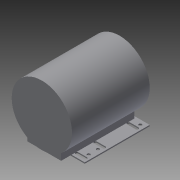
# Autodesk Inventor part: Motor4
Saved by Autodesk Inventor 2016 (Build 200138000, 138)
## iProperties
Created: 2016-02-24
Part Number: Motor4
Material: Generic
Document SubType Name: Modeling
Designer: jonesdm
Density: 1 g/cm^3
Appearance: Default
Author: jonesdm
Autodesk Inventor part; units mm, degrees
ref_plane "YZ Plane" through (0, 0, 0) normal (1, 0, 0) x (0, 1, 0)
ref_plane "XZ Plane" through (0, 0, 0) normal (0, 1, 0) x (-1, 0, 0)
ref_plane "XY Plane" through (0, 0, 0) normal (0, 0, 1) x (1, 0, 0)
sketch "Sketch1" plane through (0, 0, 0) normal (0, 0, 1) x (1, 0, 0)
  circle A0 centre (0, 0) radius 7.9375
  line L0 (-2.4257, 7.5578) -> (-2.4257, 10.0978)
  line L1 (-2.4257, 10.0978) -> (2.4257, 10.0978)
  line L2 (2.4257, 10.0978) -> (2.4257, 7.5578)
  point P0 (0, 10.0978)
  dimension "d0" = 15.875
  dimension "d1" = 2.54
  dimension "d2" = 4.8514
  constraints: 6 end point, 2 point on circle, 1 centre point, 1 coincident, 1 horizontal, 1 midpoint, 1 perpendicular, 1 vertical, 1 vertical alignment
  measures "d0" diameter of A0
  measures "d1" distance of L1.end L2.end
  measures "d2" distance of L0.end L1.end
extrude "Extrusion1" add sketch "Sketch1" along normal blind 50.8
sketch "Sketch2" plane through (0, 0, 50.8) normal (0, 0, 1) x (1, 0, 0)
  circle A0 centre (0, 0) radius 82.55
  dimension "d5" = 165.1
  constraints: 1 centre point, 1 coincident
  measures "d5" diameter of A0
extrude "Extrusion2" add sketch "Sketch2" along normal blind 212.7758
sketch "Sketch3" plane through (0, 0, 50.8) normal (0, 0, -1) x (-1, 0, 0)
  circle A0 centre (0, 0) radius 73.025
  arc A1 (-2.4257, 7.5578) -> (2.4257, 7.5578) centre (0, 0) ccw projected
  line L0 (0, 0) -> (51.6365, 51.6365)
  line L1 (0, 0) -> (73.025, 0) construction
  line L2 (0, 0) -> (51.6365, -51.6365)
  line L3 (0, 0) -> (73.025, 0) construction
  line L4 (0, 0) -> (-51.6365, 51.6365)
  line L5 (0, 0) -> (73.025, 0) construction
  line L6 (0, 0) -> (-51.6365, -51.6365)
  line L7 (0, 0) -> (73.025, 0) construction
  dimension "d8" = 146.05
  dimension "d9" = 45
  dimension "d10" = 45
  dimension "d11" = 135
  dimension "d12" = 135
  constraints: 16 end point, 5 coincident, 4 equal length, 4 horizontal, 4 point on circle, 1 centre point
  measures "d8" diameter of A0
  measures "d9" angle of L1 L0
  measures "d10" angle of L2 L3
  measures "d11" angle of L5 L4
  measures "d12" angle of L6 L7
hole "Hole1" at (51.6365, 51.6365, 50.8) at (-51.6365, 51.6365, 50.8) at (-51.6365, -51.6365, 50.8) at (51.6365, -51.6365, 50.8) direction (0, 0, 1) diameter 4.9784 depth 19.05 tip angle 118 thread size "1/4-20 UNC" class "2B" standard "ANSI Unified Screw Threads"
ref_plane "Work Plane2" through (0, -82.55, 50.8) normal (0, 1, 0) x (-1, 0, 0)
sketch "Sketch4" plane through (0, -82.55, 50.8) normal (0, 1, 0) x (-1, 0, 0)
  line L0 (82.55, 212.7758) -> (-82.55, 212.7758) projected
  line L1 (-82.55, 0) -> (82.55, 0) projected
  line L2 (82.55, 0) -> (82.55, 177.8) projected
  line L3 (-82.55, 0) -> (-82.55, 177.8) projected
  line L4 (-46.355, 6.35) -> (46.355, 6.35)
  line L5 (46.355, 6.35) -> (46.355, 206.4258)
  line L6 (46.355, 206.4258) -> (-46.355, 206.4258)
  line L7 (-46.355, 206.4258) -> (-46.355, 6.35)
  point P0 (0, -50.8)
  point P1 (0, 6.35)
  dimension "d20" = 200.0758
  dimension "d21" = 6.35
  dimension "d22" = 92.71
  constraints: 8 end point, 2 parallel, 1 horizontal, 1 midpoint, 1 perpendicular, 1 vertical alignment, 1 other
  measures "d20" distance of L4.end L5.end
  measures "d21" distance between parallel lines of L1 L4
  measures "d22" distance of L4.start L4.end
extrude "Extrusion3" add sketch "Sketch4" along normal blind 25.4 and the other way blind 5.2324
ref_plane "Work Plane7" through (0, -90.9574, 50.8) normal (0, -1, 0) x (1, 0, 0)
sketch "Sketch5" plane through (0, -90.9574, 50.8) normal (0, -1, 0) x (1, 0, 0)
  line L0 (82.55, 212.7758) -> (-82.55, 212.7758) projected
  line L1 (82.55, 212.7758) -> (-82.55, 212.7758)
  line L2 (-82.55, 212.7758) -> (-82.55, 34.9758)
  line L3 (-82.55, 34.9758) -> (82.55, 34.9758)
  line L4 (82.55, 34.9758) -> (82.55, 212.7758)
  point P0 (0, -50.8)
  dimension "d54" = 177.8
  dimension "d55" = 165.1
  constraints: 8 end point, 2 parallel, 1 horizontal, 1 perpendicular, 1 point on line
  measures "d54" distance of L1.end L2.end
  measures "d55" distance of L1.start L1.end
extrude "Extrusion4" add sketch "Sketch5" against normal blind 3.175
ref_plane "Work Plane9" through (0, -94.1324, 50.8) normal (0, -1, 0) x (1, 0, 0)
sketch "Sketch6" plane through (0, -94.1324, 50.8) normal (0, -1, 0) x (1, 0, 0)
  circle A0 centre (69.5575, 189.0141) radius 4.2291
  line L0 (73.2282, 206.0194) -> (50.3174, 206.0194)
  line L1 (50.3174, 197.5612) -> (73.2282, 197.5612)
  line L2 (77.4117, 201.1711) -> (77.4117, 202.4095)
  arc A1 (73.2282, 197.5612) -> (73.2282, 206.0194) centre (73.2282, 201.7903) ccw
  arc A2 (50.3174, 206.0194) -> (50.3174, 197.5612) centre (50.3174, 201.7903) ccw
  circle A3 centre (69.5575, 163.6903) radius 4.2291
  line L3 (73.2405, 146.685) -> (50.3297, 146.685)
  line L4 (50.3297, 155.1432) -> (73.2405, 155.1432)
  arc A4 (73.2405, 146.685) -> (73.2405, 155.1432) centre (73.2405, 150.9141) ccw
  arc A5 (50.3297, 155.1432) -> (50.3297, 146.685) centre (50.3174, 150.9141) ccw
  arc A6 (73.2405, 56.1594) -> (73.2405, 64.6176) centre (73.2405, 60.3885) ccw
  line L5 (50.3297, 56.1594) -> (73.2405, 56.1594)
  line L6 (73.2405, 64.6176) -> (50.3297, 64.6176)
  arc A7 (50.3297, 64.6176) -> (50.3297, 56.1594) centre (50.3174, 60.3885) ccw
  circle A8 centre (69.5575, 47.6123) radius 4.2291
  circle A9 centre (-69.3613, 189.0141) radius 4.2291
  line L7 (-73.0443, 206.0194) -> (-50.1335, 206.0194)
  line L8 (-50.1335, 197.5612) -> (-73.0443, 197.5612)
  line L9 (-77.2278, 201.1711) -> (-77.2278, 202.4095)
  arc A10 (-73.0443, 206.0194) -> (-73.0443, 197.5612) centre (-73.0443, 201.7903) ccw
  arc A11 (-50.1335, 197.5612) -> (-50.1335, 206.0194) centre (-50.1335, 201.7903) ccw
  arc A12 (-73.0443, 155.1432) -> (-73.0443, 146.685) centre (-73.0443, 150.9141) ccw
  line L10 (-50.1335, 155.1432) -> (-73.0443, 155.1432)
  line L11 (-73.0443, 146.685) -> (-50.1335, 146.685)
  arc A13 (-50.1335, 146.685) -> (-50.1335, 155.1432) centre (-50.1335, 150.9141) ccw
  circle A14 centre (-69.3613, 163.6903) radius 4.2291
  circle A15 centre (-69.3613, 47.6123) radius 4.2291
  line L12 (-50.1335, 56.1594) -> (-73.0443, 56.1594)
  line L13 (-73.0443, 64.6176) -> (-50.1335, 64.6176)
  arc A16 (-73.0443, 64.6176) -> (-73.0443, 56.1594) centre (-73.0443, 60.3885) ccw
  arc A17 (-50.1335, 56.1594) -> (-50.1335, 64.6176) centre (-50.1335, 60.3885) ccw
  line L14 (-82.55, 212.7758) -> (-82.55, 34.9758) projected
  line L15 (82.55, 212.7758) -> (-82.55, 212.7758) projected
  line L16 (82.55, 34.9758) -> (82.55, 212.7758) projected
  line L17 (82.55, 212.7758) -> (82.55, 34.9758) projected
  point P0 (0, -50.8)
  point P1 (-61.5889, 206.0194)
  point P2 (61.7728, 206.0194)
  point P3 (-61.5889, 197.5612)
  point P4 (61.7728, 197.5612)
  point P5 (-61.5889, 155.1432)
  point P6 (61.7851, 155.1432)
  dimension "d31" = 8.4582
  dimension "d38" = 8.4582
  dimension "d39" = 8.4582
  dimension "d40" = 22.9108
  dimension "d41" = 8.4582
  dimension "d51" = 8.5471
  dimension "d56" = 50.8762
  dimension "d57" = 12.7762
  dimension "d58" = 6.7564
  dimension "d59" = 12.7762
  dimension "d60" = 90.5256
  dimension "d62" = 9.3218
  constraints: 28 end point, 28 point on circle, 18 centre point, 11 vertical alignment, 9 horizontal alignment, 7 horizontal, 6 midpoint, 1 parallel
  measures "d31" diameter of A0
  measures "d38" diameter of A1
  measures "d39" diameter of A2
  measures "d40" distance of A2.centre A1.centre
  measures "d41" distance between parallel lines of L1 L0
  measures "d51" distance from line of L5 A8.centre
  measures "d56" distance of A10.centre A12.centre
  measures "d57" vertical distance of A12.centre A14.centre
  measures "d58" distance between parallel lines of L15 L0
  measures "d59" vertical distance of A10.centre A9.centre
  measures "d60" distance of A16.centre A12.centre
  measures "d62" distance from line of A1.centre L17
extrude "Extrusion5" cut sketch "Sketch6" against normal blind 6.35 contours A0 | A1 L2 L1 A2 L0 | A3 | L3 A5 L4 A4 | L5 A7 L6 A6 | A8 | A9 | L7 A11 L8 A10 L9 | L10 A13 L11 A12 | A14 | A15 | L12 A16 L13 A17
sketch "Sketch7" plane through (0, -87.7824, 50.8) normal (0, -1, 0) x (1, 0, 0)
  point P0 (0, -50.8)
equation "\"d3\" = ShaftL"
equation "\"d5\" = MotoD"
equation "\"d6\" = MotoL"
equation "\"ShaftL\" = 50.8"
equation "\"MotoD\" = 165.1"
equation "\"MotoL\" = 212.7758"
body "Solid1"
